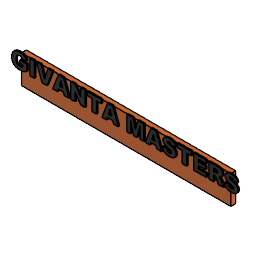
logo-strip (Autodesk Fusion 360 design; units mm, degrees)
part number: 2026-08-18-19-37-08-995
Autodesk Fusion 360 part; units mm, degrees
sketch "Sketch1" plane through (0, 0, 0) normal (0, 0, 1) x (1, 0, 0)
  line L0 (0, 0) -> (125, 0)
  line L1 (125, 0) -> (125, 3)
  line L2 (125, 3) -> (0, 3)
  line L3 (0, 3) -> (0, 0)
extrude "Extrude1" add sketch "Sketch1" along normal blind 17 makes body 1
sketch "Sketch2" plane through (0, 0, 0) normal (0, -1, 0) x (1, 0, 0)
  line L0 (0, 0) -> (125, 0)
  line L1 (125, 0) -> (125, 17)
  line L2 (125, 17) -> (0, 17)
  line L3 (0, 17) -> (0, 0)
  line L4 (8, 8.5) -> (117, 8.5)
  dimension "d151" = 9
  text T0 "GIVANTA MASTERS" font "Arial Black" height 9 align centre spacing 1 along the path L4 letters at x, y, angle (-5.6753, 22.3377, 0) (4.7981, 22.3377, 0) (9.691, 22.3377, 0) (19.4829, 22.3377, 0) (29.2995, 22.3377, 0) (39.7729, 22.3377, 0) (48.8527, 22.3377, 0) (58.6692, 22.3377, 0) (62.8622, 22.3377, 0) (74.7292, 22.3377, 0) (84.5457, 22.3377, 0) (93.6255, 22.3377, 0) (102.7053, 22.3377, 0) (111.7851, 22.3377, 0) (121.5955, 22.3377, 0)
extrude "Extrude2" add sketch "Sketch2" along normal blind 0.8 separate body text T0 makes body 2 at (104.5491, 0, 12.7708) makes body 3 at (64.5116, 0, 13.7879) makes body 4 at (26.854, 0, 12.6439) makes body 5 at (3.2551, 0, 11.7292) makes body 6 at (37.972, 0, 12.8404) makes body 7 at (82.1003, 0, 12.6439) makes body 8 at (113.6739, 0, 12.7176) makes body 9 at (97.6774, 0, 13.0184) makes body 10 at (56.2237, 0, 12.6439) makes body 11 at (12.5007, 0, 12.3411) makes body 12 at (6.7585, 0, 14.5) makes body 13 at (43.8247, 0, 13.0184) makes body 14 at (90.7117, 0, 13.219) makes body 15 at (127.7615, 0, 13.219)
equation "d152 = 'GIVANTA MASTERS'"
named bodies: "Тело", "Логотип (2-й цвет)", "Логотип", "Логотип (1)", "Логотип (2)", "Логотип (3)", "Логотип (4)", "Логотип (5)", "Логотип (6)", "Логотип (7)", "Логотип (8)", "Логотип (9)", "Логотип (10)", "Логотип (11)", "Логотип (12)"
